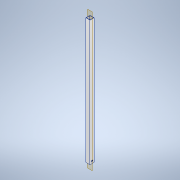
# Autodesk Inventor part: stick
Saved by Autodesk Inventor 2022 (Build 260153000, 153)
## iProperties
Created: 2022-04-20
Part Number: stick
Material: アルミニウム 6061
Document SubType Name: Modeling
Designer: Yazawa
Density: 2.7 g/cm^3
Appearance: アルミニウム - フラット
Author: Yazawa
Autodesk Inventor part; units mm, degrees
ref_plane "YZ Plane" through (0, 0, 0) normal (1, 0, 0) x (0, 1, 0)
ref_plane "XZ Plane" through (0, 0, 0) normal (0, 1, 0) x (-1, 0, 0)
sketch "スケッチ1" plane through (0, 0, 0) normal (0, 1, 0) x (-1, 0, 0)
  line L0 (5, 5) -> (-5, 5)
  line L1 (-5, 5) -> (-5, -5)
  line L2 (-5, -5) -> (5, -5)
  line L3 (5, -5) -> (5, 5)
  line L4 (4, 4) -> (-4, 4)
  line L5 (-4, 4) -> (-4, -4)
  line L6 (-4, -4) -> (4, -4)
  line L7 (4, -4) -> (4, 4)
  line L8 (5, 5) -> (-5, -5) construction
  line L9 (-5, 5) -> (5, -5) construction
  point P0 (0, 0)
  point P1 (0, 0)
  point P2 (0, 0)
  dimension "d0" = 10
  dimension "d1" = 10
  dimension "d2" = 1
  constraints: 20 end point, 4 parallel, 2 midpoint, 2 perpendicular, 1 coincident, 1 horizontal, 3 other
  measures "d0" distance of L2.end L1.end
  measures "d1" distance of L1.end L0.end
  measures "d2" distance between parallel lines of L3 L7
extrude "押し出し1" add sketch "スケッチ1" along normal blind 300
sketch "スケッチ2" plane through (5, 0, 5) normal (1, 0, 0) x (0, 0, -1)
  line L0 (0, 0) -> (10, 0) projected
  point P0 (5, 0)
  point P1 (5, 10)
  point P2 (5, 0)
  dimension "d5" = 10
  constraints: 1 coincident, 1 vertical alignment
  measures "d5" distance from line of point (5, 10) L0
hole "穴1" at (5, 10, 0) direction (-1, 0, 0) diameter 4 depth 10
ref_plane "作業平面1" through (0, 0, 5) normal (1, 0, 0) x (0, 0, -1)
sketch "スケッチ3" plane through (-5, 0, -5) normal (-1, 0, 0) x (0, 0, 1)
  line L0 (10, 0) -> (10, 300) projected
  line L1 (0, 0) -> (10, 0)
  line L2 (10, 0) -> (10, 5)
  line L3 (10, 5) -> (0, 5)
  line L4 (0, 5) -> (0, 0)
  point P0 (5, 0)
  dimension "d13" = 5
  constraints: 8 end point, 2 parallel, 1 coincident, 1 horizontal, 1 perpendicular, 1 point on line
  measures "d13" distance of L2.end L1.end
extrude "押し出し2" cut sketch "スケッチ3" against normal blind 25.4
sketch "スケッチ5" plane through (5, 300, -5) normal (0, 0, -1) x (-1, 0, 0)
  line L0 (0, -295) -> (0, 0) projected
  line L1 (0, -295) -> (10, -295) projected
  point P0 (5, -300)
  point P1 (5, -290)
  dimension "d16" = 5
  dimension "d17" = 5
  measures "d16" distance from line of L0 point (5, -290)
  measures "d17" distance from line of L1 point (5, -290)
hole "穴2" at (0, 10, -5) direction (0, 0, 1) diameter 2.459 depth 1 thread size "M3x0.5" class "6H" standard "ISO Metric profile"
ref_plane "作業平面3" through (-5, 300, 0) normal (0, 0, 1) x (1, 0, 0)
